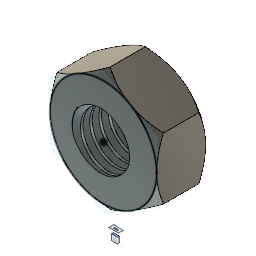
plummer block assembly by Chaitanya sharma (Autodesk Fusion 360 archive; units mm, degrees)
design "nut m10-6"
part number: 6
Autodesk Fusion 360 part; units mm, degrees
note: some values were not read from the file. Chosen so that the rebuilt part matches the saved one: which face or edge a step refers to; a direction.
sketch "Sketch1" plane through (0, 0, 0) normal (0, 1, 0) x (1, 0, 0)
  line L0 (8.6854, 4.9561) -> (0.0506, 9.9999)
  line L1 (0.0506, 9.9999) -> (-8.6348, 5.0438)
  line L2 (-8.6348, 5.0438) -> (-8.6854, -4.9561)
  line L3 (-8.6854, -4.9561) -> (-0.0506, -9.9999)
  line L4 (-0.0506, -9.9999) -> (8.6348, -5.0438)
  line L5 (8.6348, -5.0438) -> (8.6854, 4.9561)
  dimension "d1" = 10
  measures "d1" distance of L0.start L0.end
extrude "Extrude1" add sketch "Sketch1" along normal mid plane 8 makes body 1
hole "Hole1" at (0, -4, 0) direction (0, 1, 0) diameter 8.526 depth 10 tip angle 180 bodies 1
thread "Thread1" "ISO Metric profile 10.0 M10x1.5 6H" major diameter 10.198 minor diameter 8.526 pitch 1.5 angle 60 modelled right hand crest width 0.4094 on face at (0.2125, -1.3333, -4.2577) crest through (0, -3.625, -4.263) on bodies 1
sketch "Sketch2" plane through (0, -4, 0) normal (0, -1, 0) x (1, 0, 0)
  line L0 (8.6854, -4.9561) -> (8.6348, 5.0438)
  line L1 (8.6348, 5.0438) -> (-0.0506, 9.9999)
  line L2 (-0.0506, 9.9999) -> (-8.6854, 4.9561)
  line L3 (-8.6854, 4.9561) -> (-8.6348, -5.0438)
  line L4 (-8.6348, -5.0438) -> (0.0506, -9.9999)
  line L5 (0.0506, -9.9999) -> (8.6854, -4.9561)
  spline S0 degree 3 poles (2.7898, -3.2234) (2.402, -3.6309) (1.937, -3.9573) (0.8905, -4.4257) (0.3159, -4.5559) (-0.8718, -4.5934) (-1.4737, -4.4924) (-2.6259, -4.0616) (-3.1623, -3.7287) (-3.9115, -3.0347) (-4.1679, -2.7317) (-4.6081, -2.065) (-4.7886, -1.7027) (-4.9244, -1.3229) knots 0 0 0 0 0.168783 0.168783 0.343691 0.343691 0.524721 0.524721 0.711872 0.711872 0.830165 0.830165 0.950778 0.950778 0.950778 0.950778
  arc A0 (-4.9244, 1.3229) -> (-4.9244, -1.3229) centre (0, 0) ccw
  spline S1 degree 3 poles (-4.9244, 1.3229) (-4.705, 1.9366) (-4.3696, 2.5023) (-3.5118, 3.4553) (-3.0036, 3.8386) (-1.8858, 4.3764) (-1.2905, 4.5328) (-0.0939, 4.6033) (0.4953, 4.5247) (1.3844, 4.2196) (1.702, 4.0665) (2.2868, 3.6914) (2.553, 3.4722) (2.7898, 3.2234) knots 0 0 0 0 0.195529 0.195529 0.384922 0.384922 0.568175 0.568175 0.745285 0.745285 0.850991 0.850991 0.954382 0.954382 0.954382 0.954382
  arc A1 (2.7898, -3.2234) -> (2.7898, 3.2234) centre (0, 0) ccw
  circle A2 centre (0, 0) radius 8.6603
  constraint concentric A0 A2
  constraint tangent L3 A2
sketch "Sketch3" plane through (0, 0, 0) normal (1, 0, 0) x (0, 1, 0)
  line L0 (-4, 8.6603) -> (-4, -8.6603)
  line L1 (-4, 8.6603) -> (-0.7296, 12.5578)
  line L2 (-4, 8.6603) -> (0.5005, 8.6603) construction
  line L3 (-0.7296, 12.5578) -> (-4, 12.5578)
  line L4 (-4, 12.5578) -> (-4, 8.6603)
  dimension "d9" = 50
  constraint horizontal L2
  constraint coincident L0.start L1.start
  constraint horizontal L3
  measures "d9" angle of L1 L2
revolve "Revolve1" cut sketch "Sketch3" angle 360 about axis through (0, 1.75, 0) along (0, 1, 0) bodies 1
mirror "Mirror1" about plane through (0, 0, 0) normal (0, 1, 0) of "Revolve1"
copy_body "Body->Comp1" bodies 1 removing the originals makes body 2 in component "nut m10"
component "nut m10" placed x (1, 0, 0) y (0, 1, 0) z (0, 0, 1) at (0, 0, 0)

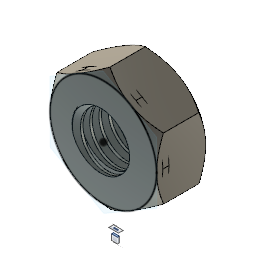
design "locknut m10-7"
part number: 7
Autodesk Fusion 360 part; units mm, degrees
sketch "Sketch1" plane through (0, 0, 0) normal (0, 1, 0) x (1, 0, 0)
  line L0 (8.6854, 4.9561) -> (0.0506, 9.9999)
  line L1 (0.0506, 9.9999) -> (-8.6348, 5.0438)
  line L2 (-8.6348, 5.0438) -> (-8.6854, -4.9561)
  line L3 (-8.6854, -4.9561) -> (-0.0506, -9.9999)
  line L4 (-0.0506, -9.9999) -> (8.6348, -5.0438)
  line L5 (8.6348, -5.0438) -> (8.6854, 4.9561)
  dimension "d1" = 10
  measures "d1" distance of L0.start L0.end
extrude "Extrude1" add sketch "Sketch1" along normal mid plane 8 makes body 1
hole "Hole1" at (0, -4, 0) direction (0, 1, 0) diameter 8.526 depth 10 tip angle 180 bodies 1
thread "Thread1" "ISO Metric profile 10.0 M10x1.5 6H" major diameter 10.198 minor diameter 8.526 pitch 1.5 angle 60 modelled right hand crest width 0.4094 on face at (0.2125, -1.3333, -4.2577) crest through (0, -3.625, -4.263) on bodies 1
sketch "Sketch2" plane through (0, -4, 0) normal (0, -1, 0) x (1, 0, 0)
  line L0 (8.6854, -4.9561) -> (8.6348, 5.0438)
  line L1 (8.6348, 5.0438) -> (-0.0506, 9.9999)
  line L2 (-0.0506, 9.9999) -> (-8.6854, 4.9561)
  line L3 (-8.6854, 4.9561) -> (-8.6348, -5.0438)
  line L4 (-8.6348, -5.0438) -> (0.0506, -9.9999)
  line L5 (0.0506, -9.9999) -> (8.6854, -4.9561)
  spline S0 degree 3 poles (2.7898, -3.2234) (2.402, -3.6309) (1.937, -3.9573) (0.8905, -4.4257) (0.3159, -4.5559) (-0.8718, -4.5934) (-1.4737, -4.4924) (-2.6259, -4.0616) (-3.1623, -3.7287) (-3.9115, -3.0347) (-4.1679, -2.7317) (-4.6081, -2.065) (-4.7886, -1.7027) (-4.9244, -1.3229) knots 0 0 0 0 0.168783 0.168783 0.343691 0.343691 0.524721 0.524721 0.711872 0.711872 0.830165 0.830165 0.950778 0.950778 0.950778 0.950778
  arc A0 (-4.9244, 1.3229) -> (-4.9244, -1.3229) centre (0, 0) ccw
  spline S1 degree 3 poles (-4.9244, 1.3229) (-4.705, 1.9366) (-4.3696, 2.5023) (-3.5118, 3.4553) (-3.0036, 3.8386) (-1.8858, 4.3764) (-1.2905, 4.5328) (-0.0939, 4.6033) (0.4953, 4.5247) (1.3844, 4.2196) (1.702, 4.0665) (2.2868, 3.6914) (2.553, 3.4722) (2.7898, 3.2234) knots 0 0 0 0 0.195529 0.195529 0.384922 0.384922 0.568175 0.568175 0.745285 0.745285 0.850991 0.850991 0.954382 0.954382 0.954382 0.954382
  arc A1 (2.7898, -3.2234) -> (2.7898, 3.2234) centre (0, 0) ccw
  circle A2 centre (0, 0) radius 8.6603
  constraint concentric A0 A2
  constraint tangent L3 A2
sketch "Sketch3" plane through (0, 0, 0) normal (1, 0, 0) x (0, 1, 0)
  line L0 (-4, 8.6603) -> (-4, -8.6603)
  line L1 (-4, 8.6603) -> (-0.7296, 12.5578)
  line L2 (-4, 8.6603) -> (0.5005, 8.6603) construction
  line L3 (-0.7296, 12.5578) -> (-4, 12.5578)
  line L4 (-4, 12.5578) -> (-4, 8.6603)
  dimension "d9" = 50
  constraint horizontal L2
  constraint coincident L0.start L1.start
  constraint horizontal L3
  measures "d9" angle of L1 L2
revolve "Revolve1" cut sketch "Sketch3" angle 360 about axis through (0, 1.75, 0) along (0, 1, 0) bodies 1
mirror "Mirror1" about plane through (0, 0, 0) normal (0, 1, 0) of "Revolve1"
copy_body "Body->Comp1" bodies 1 removing the originals makes body 2 in component "locknut m10"
extrude "Extrude1'" cut 1 faces at (6.9934, -4, 1.6188) along direction (0, -1, 0) blind -1 and the other way blind 2 on bodies 2 bodies 2 in component "locknut m10"
component "locknut m10" placed x (1, 0, 0) y (0, 1, 0) z (0, 0, 1) at (0, 0, 0)

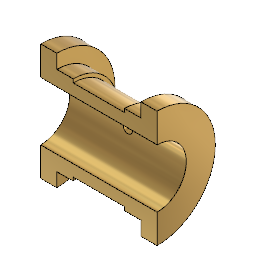
design "bearing top half"
part number: 4
Autodesk Fusion 360 part; units mm, degrees
sketch "Sketch1" plane through (0, 0, 0) normal (0, 1, 0) x (1, 0, 0)
  line L0 (25, -12.5) -> (25, -25)
  line L1 (25, -25) -> (18, -25)
  line L2 (18, -25) -> (18, -19)
  line L3 (18, -19) -> (11, -19)
  line L4 (11, -19) -> (11, -17.5)
  line L5 (11, -17.5) -> (0, -17.5)
  line L6 (0, -12.5) -> (25, -12.5)
  line L7 (-18, -25) -> (-18, -19)
  line L8 (0, -12.5) -> (-25, -12.5)
  line L9 (-25, -12.5) -> (-25, -25)
  line L10 (-11, -19) -> (-11, -17.5)
  line L11 (-11, -17.5) -> (0, -17.5)
  line L12 (-18, -19) -> (-11, -19)
  line L13 (-25, -25) -> (-18, -25)
  dimension "d3" = 18
  dimension "d4" = 6
  dimension "d5" = 11
  dimension "d6" = 1.5
  constraint perpendicular L0 L1
  constraint perpendicular L1 L2
  constraint perpendicular L2 L3
  constraint perpendicular L3 L4
  constraint perpendicular L4 L5
  measures "d3" horizontal distance of origin L1.end
  measures "d4" distance of L1.end L2.end
  measures "d5" horizontal distance of origin L3.end
  measures "d6" distance of L3.end L4.end
revolve "Revolve1" add sketch "Sketch1" angle 180 about axis through (1.75, 0, 0) along (-1, 0, 0) makes body 1
sketch "Sketch2" plane through (0, 0, 0) normal (0, 1, 0) x (1, 0, 0)
  circle A0 centre (0, 0) radius 2
  dimension "d9" = 4
  constraint coincident A0.centre origin
  measures "d9" diameter of A0
extrude "Extrude1" cut sketch "Sketch2" along normal blind 28 bodies 1
copy_body "Body->Comp1" bodies 1 removing the originals makes body 2 in component "bearing top half"
component "bearing top half" placed x (1, 0, 0) y (0, 1, 0) z (0, 0, 1) at (0, 0, 0)
